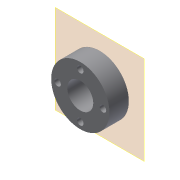
# Autodesk Inventor part: Spacer
Saved by Autodesk Inventor 2017 (Build 210142000, 142)
## iProperties
Created: 2016-07-28
Part Number: Spacer
Material: Generic
Document SubType Name: Modeling
Designer: Tutorial Books
Density: 1 g/cm^3
Appearance: Default
Author: Tutorial Books
Autodesk Inventor part; units mm, degrees
ref_plane "YZ Plane" through (0, 0, 0) normal (1, 0, 0) x (0, 1, 0)
ref_plane "XZ Plane" through (0, 0, 0) normal (0, 1, 0) x (-1, 0, 0)
ref_plane "XY Plane" through (0, 0, 0) normal (0, 0, 1) x (1, 0, 0)
ref_plane "Work Plane1" through (0, 0, 0) normal (0, 0, 1) x (1, 0, 0)
sketch "Sketch1" plane through (0, 0, 0) normal (0, 0, 1) x (1, 0, 0)
  circle A0 centre (44.45, 0) radius 6.35 projected
  circle A1 centre (0, -44.45) radius 6.35 projected
  circle A2 centre (-44.45, 0) radius 6.35 projected
  circle A3 centre (0, 44.45) radius 6.35 projected
  circle A4 centre (0, 0) radius 25.4 projected
  circle A5 centre (0, 0) radius 57.15
  point P0 (0, 0)
  dimension "d0" = 114.3
  constraints: 1 centre point, 1 coincident
  measures "d0" diameter of A5
extrude "Extrusion1" add sketch "Sketch1" along normal blind 38.1
body "Solid1"
